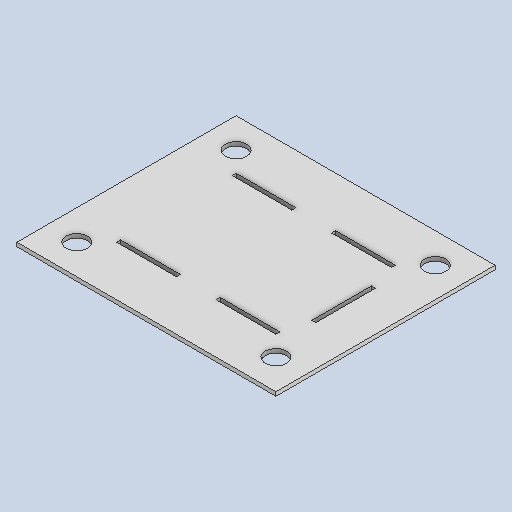
# Autodesk Inventor part: bottom_hinge_001
Saved by Autodesk Inventor 2025.2 (Build 292293000, 293)
## iProperties
Created: 2025-03-24
Part Number: bottom_hinge_001
Material: Generic
Document SubType Name: Sheet Metal
Designer: Caspe
Density: 1 g/cm^3
Sheet Metal Rule: Default_mm
Appearance: Default
Author: Caspe
Autodesk Inventor part; units mm, degrees
ref_plane "YZ Plane" through (0, 0, 0) normal (1, 0, 0) x (0, 1, 0)
ref_plane "XZ Plane" through (0, 0, 0) normal (0, 1, 0) x (-1, 0, 0)
ref_plane "XY Plane" through (0, 0, 0) normal (0, 0, 1) x (1, 0, 0)
sketch "Sketch1" plane through (0, 0, 0) normal (0, 1, 0) x (-1, 0, 0)
  line L0 (0, 0) -> (-130, 0)
  line L1 (-130, 0) -> (-130, -110)
  line L2 (-130, -110) -> (0, -110)
  line L3 (0, -110) -> (0, 0)
  circle A0 centre (-15, -95) radius 5.35
  line L4 (-65, -110) -> (-65, 0)
  line L5 (0, -55) -> (-130, -55)
  circle A1 centre (-115, -95) radius 5.35
  circle A2 centre (-15, -15) radius 5.35
  circle A3 centre (-115, -15) radius 5.35
  dimension "d0" = 130
  dimension "d1" = 110
  dimension "d2" = 10.7
  dimension "d3" = 50
  dimension "d4" = 40
  measures "d0" distance of L2.end L1.end
  measures "d1" distance of L1.end L0.end
  measures "d2" diameter of A0
  measures "d3" distance from line of L4 A0.centre
  measures "d4" distance from line of L5 A0.centre
extrude "Plate1" add sketch "Sketch1" along normal blind 2
sketch "Sketch2" plane through (0, 2, 0) normal (0, 1, 0) x (1, 0, 0)
  line L0 (0, 110) -> (0, 0) projected
  line L1 (0, 55) -> (130, 55)
  line L2 (130, 0) -> (130, 110) projected
  line L3 (25, 85) -> (55, 85)
  line L4 (55, 85) -> (55, 83)
  line L5 (55, 83) -> (25, 83)
  line L6 (25, 83) -> (25, 85)
  line L7 (75, 83) -> (105, 83)
  line L8 (105, 83) -> (105, 85)
  line L9 (105, 85) -> (75, 85)
  line L10 (75, 85) -> (75, 83)
  line L11 (108, 55) -> (110, 55)
  line L12 (110, 55) -> (110, 70)
  line L13 (110, 70) -> (108, 70)
  line L14 (108, 70) -> (108, 55)
  line L15 (25, 25) -> (55, 25)
  line L16 (55, 25) -> (55, 27)
  line L17 (55, 27) -> (25, 27)
  line L18 (25, 27) -> (25, 25)
  line L19 (75, 27) -> (105, 27)
  line L20 (105, 27) -> (105, 25)
  line L21 (105, 25) -> (75, 25)
  line L22 (75, 25) -> (75, 27)
  line L23 (110, 55) -> (110, 40)
  line L24 (110, 40) -> (108, 40)
  line L25 (108, 40) -> (108, 55)
  point P0 (75, 84)
  point P1 (55, 84)
  dimension "d6" = 2
  dimension "d7" = 30
  dimension "d8" = 30
  dimension "d9" = 2
  dimension "d10" = 2
  dimension "d11" = 15
  dimension "d12" = 20
  dimension "d13" = 25
  dimension "d14" = 20
  dimension "d15" = 28
  constraints: 48 end point, 10 symmetric about line, 6 parallel, 4 midpoint, 3 horizontal, 3 perpendicular, 1 collinear, 1 point on line
  measures "d6" distance between parallel lines of L3 L5
  measures "d7" distance between parallel lines of L4 L6
  measures "d8" distance of L9.end L8.end
  measures "d9" distance of L8.end L7.end
  measures "d10" distance of L13.end L12.end
  measures "d11" distance between parallel lines of L1 L13
  measures "d12" distance of point (75, 84) point (55, 84)
  measures "d13" distance between parallel lines of L2 L8
  measures "d14" distance between parallel lines of L2 L12
  measures "d15" distance between parallel lines of L1 L7
extrude "Cut1" cut sketch "Sketch2" against normal blind 2
equation "\"d6\" = plate_thickness"
equation "\"d9\" = plate_thickness"
equation "\"d10\" = plate_thickness"
equation "\"d16\" = Thickness"
equation "\"d5\" = Thickness"
equation "\"BendRadius\" = Thickness"
equation "\"BendReliefWidth\" = Thickness"
equation "\"BendReliefDepth\" = 0.5 * Thickness"
equation "\"CornerReliefSize\" = 4 * Thickness"
equation "\"MinimumRemnant\" = 2 * Thickness"
equation "\"TransitionRadius\" = BendRadius"
equation "\"JacobiRadiusSize\" = BendRadius"
equation "\"GapSize\" = Thickness"
equation "\"l___________\" = 0"
equation "\"l__________\" = 0"
equation "\"l_________\" = 0"
equation "\"rivet_diameter\" = 4"
equation "\"plate_thickness\" = 2"
equation "\"l________\" = 0"
equation "\"A_joint_tolerance\" = 3"
equation "\"A_B_spacing\" = 2"
equation "\"Thickness\" = 2"
body "Solid1"
